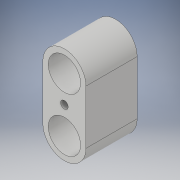
# Autodesk Inventor part: BearingIn
Saved by Autodesk Inventor 2019 (Build 230136000, 136)
## iProperties
Created: 2021-01-03
Part Number: BearingIn
Material: Типовые
Document SubType Name: Modeling
Designer: Professional
Density: 1 g/cm^3
Appearance: По умолчанию
Author: Professional
Autodesk Inventor part; units mm, degrees
ref_plane "YZ Plane" through (0, 0, 0) normal (1, 0, 0) x (0, 1, 0)
ref_plane "XZ Plane" through (0, 0, 0) normal (0, 1, 0) x (-1, 0, 0)
ref_plane "XY Plane" through (0, 0, 0) normal (0, 0, 1) x (1, 0, 0)
sketch "Эскиз1" plane through (0, 0, 0) normal (0, 0, 1) x (1, 0, 0)
  circle A0 centre (0, 10) radius 6
  circle A1 centre (0, -10) radius 6
  line L0 (0, -10) -> (0, 10) construction
  line L1 (8, -10) -> (8, 10)
  line L2 (-8, 10) -> (-8, -10)
  arc A2 (-8, -10) -> (8, -10) centre (0, -10) ccw
  arc A3 (8, 10) -> (-8, 10) centre (0, 10) ccw
  circle A4 centre (0, 0) radius 1.4
  dimension "d0" = 12
  dimension "d1" = 8
  dimension "d2" = 20
  dimension "d5" = 2.8
  constraints: 8 end point, 5 centre point, 4 point on circle, 4 tangent, 2 coincident, 1 equal radius, 1 midpoint, 1 parallel, 1 vertical
  measures "d0" diameter of A0
  measures "d1" radius of A3
  measures "d2" distance of L0.start L0.end
  measures "d5" diameter of A4
extrude "Выдавливание1" add sketch "Эскиз1" along normal blind 19
